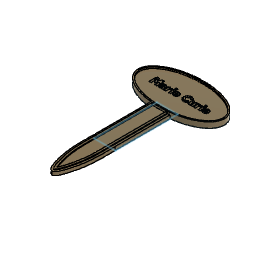
Rosen-Tafel_Marie_Curie v2 (Autodesk Fusion 360 design; units mm, degrees)
Autodesk Fusion 360 part; units mm, degrees
sketch "Skizze1" plane through (0, 0, 0) normal (0, 0, 1) x (1, 0, 0) in component "Tafe"
  ellipse E0 centre (0, 0) end of major axis (60, 0) minor radius 30
  line L0 (-60, 0) -> (60, 0)
  line L1 (0, -30) -> (0, 30)
  dimension "d1" = 60
  constraint coincident E0.centre origin
  constraint horizontal L0
  constraint coincident E0 L0.start
  constraint coincident E0 L0.end
  constraint coincident E0 L1.start
  constraint coincident E0 L1.end
  measures "d1" distance of E0
extrude "Extrusion1" add sketch "Skizze1" along normal blind 3 makes body 1 in component "Tafe"
sketch "Skizze2" plane through (0, 0, 3) normal (0, 0, 1) x (-1, 0, 0) in component "Tafe"
  ellipse E0 centre (0, 0) end of major axis (-60, 0) minor radius 30
  spline S0 degree 3 poles (61.9509, 0) (61.9509, 4.2635) (60.3055, 8.4828) (57.3091, 12.2636) (52.6449, 18.1488) (44.7166, 23.0684) (34.8255, 26.4973) (25.2136, 29.8294) (13.7584, 31.7256) (2.1658, 31.9316) (-9.8896, 32.1459) (-22.0459, 30.5274) (-32.3487, 27.3124) (-41.3637, 24.4992) (-48.9522, 20.4892) (-54.1681, 15.6411) (-58.1005, 11.9859) (-60.7028, 7.8251) (-61.5993, 3.4465) (-62.4053, -0.4903) (-61.7899, -4.5541) (-59.8722, -8.3093) (-56.3973, -15.1137) (-48.7697, -20.9418) (-38.5998, -25.0786) (-29.6788, -28.7075) (-18.796, -31.0188) (-7.5068, -31.7189) (4.0223, -32.434) (15.9353, -31.462) (26.4461, -28.9362) (36.7725, -26.4548) (45.7187, -22.4959) (52.0049, -17.4981) (56.4978, -13.926) (59.6597, -9.8063) (61.0885, -5.3839) (61.6588, -3.6187) (61.9509, -1.8099) (61.9509, 0) knots -3.141593 -3.141593 -3.141593 -3.141593 -2.764311 -2.764311 -2.764311 -2.177028 -2.177028 -2.177028 -1.606323 -1.606323 -1.606323 -1.012833 -1.012833 -1.012833 -0.49353 -0.49353 -0.49353 -0.102016 -0.102016 -0.102016 0.249996 0.249996 0.249996 0.887852 0.887852 0.887852 1.447382 1.447382 1.447382 2.018805 2.018805 2.018805 2.580199 2.580199 2.580199 2.981436 2.981436 2.981436 3.141593 3.141593 3.141593 3.141593
  dimension "d4" = 1.9509
extrude "Extrusion2" add sketch "Skizze2" along normal blind 2 and the other way blind 2 bodies 1 in component "Tafe"
sketch "Skizze3" plane through (0, 0, 0) normal (0, 0, 1) x (1, 0, 0) in component "Tafe"
extrude "Extrusion3" add 1 faces at (23.0091, -28.1834, 1) along direction (0, 0, -1) blind 1 on bodies 1 bodies 1 in component "Tafe"
sketch "Skizze1 (2)" plane through (0, 0, 0) normal (0, 0, 1) x (1, 0, 0) in component "Ständer"
extrude "Extrusion4" add 2 faces at (23.0091, -28.1834, 0) (8.4972, -9.7981, 0) along direction (0, 0, -1) blind 3 on bodies 1 bodies 1 in component "Tafe"
sketch "Skizze2 (2)" plane through (0, 0, -3) normal (0, 0, -1) x (1, 0, 0) in component "Ständer"
  spline S0 degree 3 poles (-61.9509, 0) (-61.9509, -1.8099) (-61.6588, -3.6187) (-61.0885, -5.3839) (-59.6597, -9.8063) (-56.4978, -13.926) (-52.0049, -17.4981) (-45.7187, -22.4959) (-36.7725, -26.4548) (-26.4461, -28.9362) (-15.9353, -31.462) (-4.0223, -32.434) (7.5068, -31.7189) (18.796, -31.0188) (29.6788, -28.7075) (38.5998, -25.0786) (48.7697, -20.9418) (56.3973, -15.1137) (59.8722, -8.3093) (61.7899, -4.5541) (62.4053, -0.4903) (61.5993, 3.4465) (60.7028, 7.8251) (58.1005, 11.9859) (54.1681, 15.6411) (48.9522, 20.4892) (41.3637, 24.4992) (32.3487, 27.3124) (22.0459, 30.5274) (9.8896, 32.1459) (-2.1658, 31.9316) (-13.7584, 31.7256) (-25.2136, 29.8294) (-34.8255, 26.4973) (-44.7166, 23.0684) (-52.6449, 18.1488) (-57.3091, 12.2636) (-60.3055, 8.4828) (-61.9509, 4.2635) (-61.9509, 0) knots -3.141593 -3.141593 -3.141593 -3.141593 -2.981436 -2.981436 -2.981436 -2.580199 -2.580199 -2.580199 -2.018805 -2.018805 -2.018805 -1.447382 -1.447382 -1.447382 -0.887852 -0.887852 -0.887852 -0.249996 -0.249996 -0.249996 0.102016 0.102016 0.102016 0.49353 0.49353 0.49353 1.012833 1.012833 1.012833 1.606323 1.606323 1.606323 2.177028 2.177028 2.177028 2.764311 2.764311 2.764311 3.141593 3.141593 3.141593 3.141593
  line L0 (15, 20) -> (-15, 20)
  line L1 (-15, 20) -> (-15, 110)
  line L2 (-15, 110) -> (15, 110)
  line L3 (15, 110) -> (15, 20)
  constraint horizontal L0
  constraint vertical L1
  constraint horizontal L2
  constraint vertical L3
extrude "Extrusion1'" add sketch "Skizze2 (2)" against normal blind 5 separate body contours S0 L0 L1 L3 picked at (1.6815, 23.9477) makes body 2 in component "Ständer"
extrude "Extrusion2'" add sketch "Skizze2 (2)" against normal blind 5 contours S0 L1 L2 L3 bodies 2 in component "Ständer"
sketch "Skizze3 (2)" plane through (0, 0, 2) normal (0, 0, 1) x (-1, 0, 0) in component "Ständer"
  line L0 (15, 20) -> (15, 110)
  line L1 (15, 110) -> (-15, 110)
  line L2 (-15, 110) -> (-15, 20)
  line L3 (-15, 20) -> (15, 20)
  spline S0 degree 5 poles (15, 110) (15.0176, 110.8619) (15.0503, 112.5708) (15.0915, 115.0899) (15.1309, 118.3598) (15.1537, 122.2987) (15.1484, 126.0898) (15.1122, 129.7366) (15.0406, 133.2467) (14.9275, 136.6331) (14.7639, 139.9163) (14.5397, 143.1226) (14.2439, 146.2818) (13.867, 149.4242) (13.4012, 152.5784) (12.8426, 155.769) (12.1915, 159.0132) (11.4507, 162.3163) (10.6251, 165.6668) (9.72, 169.0317) (8.7408, 172.3517) (7.6913, 175.5347) (6.574, 178.4677) (5.3908, 181.0335) (4.1426, 183.1253) (2.8302, 184.6621) (1.7296, 185.4171) (0.8758, 185.7125) (0.294, 185.7893) (0, 185.7977) knots 0 0 0 0 0 0 0.04 0.08 0.12 0.16 0.2 0.24 0.28 0.32 0.36 0.4 0.44 0.48 0.52 0.56 0.6 0.64 0.68 0.72 0.76 0.8 0.84 0.88 0.92 0.96 1 1 1 1 1 1
  line L4 (0, -2.5) -> (0, -20)
  spline S1 degree 5 poles (-15, 110) (-15.0176, 110.8619) (-15.0503, 112.5708) (-15.0915, 115.0899) (-15.1309, 118.3598) (-15.1537, 122.2987) (-15.1484, 126.0898) (-15.1122, 129.7366) (-15.0406, 133.2467) (-14.9275, 136.6331) (-14.7639, 139.9163) (-14.5397, 143.1226) (-14.2439, 146.2818) (-13.867, 149.4242) (-13.4012, 152.5784) (-12.8426, 155.769) (-12.1915, 159.0132) (-11.4507, 162.3163) (-10.6251, 165.6668) (-9.72, 169.0317) (-8.7408, 172.3517) (-7.6913, 175.5347) (-6.574, 178.4677) (-5.3908, 181.0335) (-4.1426, 183.1253) (-2.8302, 184.6621) (-1.7296, 185.4171) (-0.8758, 185.7125) (-0.294, 185.7893) (0, 185.7977) knots 0 0 0 0 0 0 0.04 0.08 0.12 0.16 0.2 0.24 0.28 0.32 0.36 0.4 0.44 0.48 0.52 0.56 0.6 0.64 0.68 0.72 0.76 0.8 0.84 0.88 0.92 0.96 1 1 1 1 1 1
  line L5 (14.8117, 100.8471) -> (15.1883, 119.1529)
  line L6 (6.7737, 185.6047) -> (-6.7737, 185.9906)
  line L7 (-14.8117, 100.8471) -> (-15.1883, 119.1529)
  line L8 (-6.7737, 185.6047) -> (6.7737, 185.9906)
  point P0 (15, 134.2579)
  point P1 (13.5579, 151.4378)
  point P2 (9.54, 169.5876)
  point P3 (3.9981, 183.1652)
  point P4 (-15, 134.2579)
  point P5 (-13.5579, 151.4378)
  point P6 (-9.54, 169.5876)
  point P7 (-3.9981, 183.1652)
  constraint coincident L0.end L1.start
  constraint midpoint L0.end L5
  constraint midpoint S0.end L6
  constraint symmetric L0.end L4 L1.end
  constraint symmetric P0 L4 P4
  constraint symmetric P1 L4 P5
  constraint symmetric P2 L4 P6
  constraint symmetric P3 L4 P7
  constraint symmetric S0.end L4 S1.end
  constraint symmetric L4 L5.start L7.start
  constraint symmetric L4 L5.end L7.end
  constraint symmetric L4 L6.start L8.start
  constraint symmetric L4 L6.end L8.end
extrude "Extrusion3'" add sketch "Skizze3 (2)" against normal blind 5 contours L1 S0 S1 bodies 2 in component "Ständer"
sketch "Skizze4" plane through (0, 0, 2) normal (0, 0, 1) x (-1, 0, 0) in component "Ständer"
  line L0 (15, 20) -> (15, 110)
  spline S0 degree 5 poles (15, 110) (15.0176, 110.8619) (15.0503, 112.5708) (15.0915, 115.0899) (15.1309, 118.3598) (15.1537, 122.2987) (15.1484, 126.0898) (15.1122, 129.7366) (15.0406, 133.2467) (14.9275, 136.6331) (14.7639, 139.9163) (14.5397, 143.1226) (14.2439, 146.2818) (13.867, 149.4242) (13.4012, 152.5784) (12.8426, 155.769) (12.1915, 159.0132) (11.4507, 162.3163) (10.6251, 165.6668) (9.72, 169.0317) (8.7408, 172.3517) (7.6913, 175.5347) (6.574, 178.4677) (5.3908, 181.0335) (4.1426, 183.1253) (2.8302, 184.6621) (1.7296, 185.4171) (0.8758, 185.7125) (0.294, 185.7893) (0, 185.7977) knots 0 0 0 0 0 0 0.04 0.08 0.12 0.16 0.2 0.24 0.28 0.32 0.36 0.4 0.44 0.48 0.52 0.56 0.6 0.64 0.68 0.72 0.76 0.8 0.84 0.88 0.92 0.96 1 1 1 1 1 1
  spline S1 degree 5 poles (-15, 110) (-15.0176, 110.8619) (-15.0503, 112.5708) (-15.0915, 115.0899) (-15.1309, 118.3598) (-15.1537, 122.2987) (-15.1484, 126.0898) (-15.1122, 129.7366) (-15.0406, 133.2467) (-14.9275, 136.6331) (-14.7639, 139.9163) (-14.5397, 143.1226) (-14.2439, 146.2818) (-13.867, 149.4242) (-13.4012, 152.5784) (-12.8426, 155.769) (-12.1915, 159.0132) (-11.4507, 162.3163) (-10.6251, 165.6668) (-9.72, 169.0317) (-8.7408, 172.3517) (-7.6913, 175.5347) (-6.574, 178.4677) (-5.3908, 181.0335) (-4.1426, 183.1253) (-2.8302, 184.6621) (-1.7296, 185.4171) (-0.8758, 185.7125) (-0.294, 185.7893) (0, 185.7977) knots 0 0 0 0 0 0 0.04 0.08 0.12 0.16 0.2 0.24 0.28 0.32 0.36 0.4 0.44 0.48 0.52 0.56 0.6 0.64 0.68 0.72 0.76 0.8 0.84 0.88 0.92 0.96 1 1 1 1 1 1
  line L1 (-15, 110) -> (-15, 20)
  line L2 (-15, 20) -> (15, 20)
  spline S2 degree 3 poles (-11.9777, 110.0309) (-11.9779, 110.0412) (-11.9781, 110.0515) (-11.9783, 110.0618) (-12.1467, 118.2962) (-12.1876, 125.6884) (-12.0304, 132.2915) (-11.8915, 138.1249) (-11.5879, 143.3276) (-10.915, 148.5264) (-10.4464, 152.1476) (-9.7926, 155.8041) (-8.949, 159.6156) (-8.1726, 163.1233) (-7.2391, 166.7794) (-6.1929, 170.2595) (-5.0109, 174.1918) (-3.6533, 177.8638) (-2.3593, 180.1318) (-1.7058, 181.2772) (-1.0734, 182.0403) (-0.6357, 182.4064) (-0.297, 182.6897) (-0.1153, 182.7456) (0, 182.7673) knots -0.000287 -0.000287 -0.000287 -0.000287 0 0 0 0.23016 0.23016 0.23016 0.433487 0.433487 0.433487 0.575116 0.575116 0.575116 0.705456 0.705456 0.705456 0.852728 0.852728 0.852728 0.927106 0.927106 0.927106 0.984664 0.984664 0.984664 0.984664
  spline S3 degree 3 poles (11.9777, 110.0309) (11.9779, 110.0412) (11.9781, 110.0515) (11.9783, 110.0618) (12.1467, 118.2962) (12.1876, 125.6884) (12.0304, 132.2915) (11.8915, 138.1249) (11.5879, 143.3276) (10.915, 148.5264) (10.4464, 152.1476) (9.7926, 155.8041) (8.949, 159.6156) (8.1726, 163.1233) (7.2391, 166.7794) (6.1929, 170.2595) (5.0109, 174.1918) (3.6533, 177.8638) (2.3593, 180.1318) (1.7058, 181.2772) (1.0734, 182.0403) (0.6357, 182.4064) (0.297, 182.6897) (0.1153, 182.7456) (0, 182.7673) knots -0.000287 -0.000287 -0.000287 -0.000287 0 0 0 0.23016 0.23016 0.23016 0.433487 0.433487 0.433487 0.575116 0.575116 0.575116 0.705456 0.705456 0.705456 0.852728 0.852728 0.852728 0.927106 0.927106 0.927106 0.984664 0.984664 0.984664 0.984664
  line L3 (11.9777, 23.0223) -> (11.9777, 110.0309)
  line L4 (-11.9777, 23.0223) -> (11.9777, 23.0223)
  line L5 (-11.9777, 110.0309) -> (-11.9777, 23.0223)
  spline S4 degree 3 poles (-9, 110.0613) (-9.0004, 110.0818) (-9.0008, 110.1022) (-9.0013, 110.1226) (-9.1708, 118.4153) (-9.2103, 125.8461) (-9.0484, 132.4316) (-8.9146, 137.8751) (-8.6346, 142.7164) (-8.0427, 147.5055) (-7.6174, 150.9474) (-7.0241, 154.4041) (-6.2475, 158.0272) (-5.5493, 161.2843) (-4.705, 164.6878) (-3.7598, 167.9778) (-2.8347, 171.1978) (-1.801, 174.2968) (-0.8034, 176.5706) (-0.5276, 177.1992) (-0.2561, 177.763) (0, 178.2439) knots -0.000569 -0.000569 -0.000569 -0.000569 0 0 0 0.232641 0.232641 0.232641 0.424939 0.424939 0.424939 0.56314 0.56314 0.56314 0.687378 0.687378 0.687378 0.80897 0.80897 0.80897 0.842587 0.842587 0.842587 0.842587
  spline S5 degree 3 poles (9, 110.0613) (9.0004, 110.0818) (9.0008, 110.1022) (9.0013, 110.1226) (9.1708, 118.4153) (9.2103, 125.8461) (9.0484, 132.4316) (8.9146, 137.8751) (8.6346, 142.7164) (8.0427, 147.5055) (7.6174, 150.9474) (7.0241, 154.4041) (6.2475, 158.0272) (5.5493, 161.2843) (4.705, 164.6878) (3.7598, 167.9778) (2.8347, 171.1978) (1.801, 174.2968) (0.8034, 176.5706) (0.5276, 177.1992) (0.2561, 177.763) (0, 178.2439) knots -0.000569 -0.000569 -0.000569 -0.000569 0 0 0 0.232641 0.232641 0.232641 0.424939 0.424939 0.424939 0.56314 0.56314 0.56314 0.687378 0.687378 0.687378 0.80897 0.80897 0.80897 0.842587 0.842587 0.842587 0.842587
  line L6 (9, 26) -> (9, 110.0613)
  line L7 (-9, 26) -> (9, 26)
  line L8 (-9, 110.0613) -> (-9, 26)
  dimension "d19" = -3.0223
  dimension "d20" = -6
extrude "Extrusion4'" add sketch "Skizze4" along normal blind 1 contours S2 S3 L3 L4 L5 bodies 2 in component "Ständer"
combine "Kombinieren1" operation add target body 1 tool bodies 2 in component "Tafe"
sketch "Skizze1 (3)" plane through (0, 0, 3) normal (0, 0, 1) x (-1, 0, 0)
  ellipse E0 centre (0, 0) end of major axis (-60, 0) minor radius 30
  line L0 (37.6827, 1.5082) -> (37.6827, 5.3738)
  line L1 (37.6827, 5.3738) -> (40.7098, 5.3738)
  line L2 (40.7098, 5.3738) -> (40.7098, -3.8782)
  line L3 (40.7098, -3.8782) -> (37.6827, 1.5082)
  line L4 (40.2977, -5.6262) -> (37.2095, -5.6262)
  line L5 (37.2095, -5.6262) -> (35.1032, -1.4621)
  line L6 (35.1032, -1.4621) -> (32.8833, -5.6262)
  line L7 (32.8833, -5.6262) -> (29.4256, -5.6262)
  line L8 (29.4256, -5.6262) -> (29.4256, 5.3738)
  line L9 (29.4256, 5.3738) -> (32.5238, 5.3738)
  line L10 (32.5238, 5.3738) -> (32.5238, -1.0074)
  line L11 (32.5238, -1.0074) -> (35.1032, 3.5831)
  line L12 (35.1032, 3.5831) -> (40.2977, -5.6262)
  spline S0 degree 2 poles (25.56, -0.4105) (26.3132, -0.3536) (26.7822, -0.2044) knots 0 0 0 1 1 1
  spline S1 degree 2 poles (26.7822, -0.2044) (27.2512, -0.0552) (27.5354, 0.1012) knots 0 0 0 1 1 1
  line L13 (27.5354, 0.1012) -> (28.2602, -1.6753)
  spline S2 degree 2 poles (28.2602, -1.6753) (27.8481, -1.8743) (27.2156, -2.0519) knots 0 0 0 1 1 1
  spline S3 degree 2 poles (27.2156, -2.0519) (26.5832, -2.2296) (25.56, -2.3148) knots 0 0 0 1 1 1
  line L14 (25.56, -2.3148) -> (25.56, -0.4105)
  spline S4 degree 2 poles (24.7214, 1.9771) (25.2899, 1.9914) (25.6168, 2.2543) knots 0 0 0 1 1 1
  spline S5 degree 2 poles (25.6168, 2.2543) (25.9437, 2.5172) (25.9437, 2.972) knots 0 0 0 1 1 1
  spline S6 degree 2 poles (25.9437, 2.972) (25.9437, 3.4125) (25.5671, 3.6186) knots 0 0 0 1 1 1
  spline S7 degree 2 poles (25.5671, 3.6186) (25.1904, 3.8247) (24.7214, 3.8389) knots 0 0 0 1 1 1
  line L15 (24.7214, 3.8389) -> (24.7214, 5.388)
  spline S8 degree 2 poles (24.7214, 5.388) (24.9631, 5.4591) (25.2331, 5.5017) knots 0 0 0 1 1 1
  spline S9 degree 2 poles (25.2331, 5.5017) (25.5031, 5.5443) (25.83, 5.5443) knots 0 0 0 1 1 1
  spline S10 degree 2 poles (25.83, 5.5443) (26.4553, 5.5443) (26.9882, 5.3596) knots 0 0 0 1 1 1
  spline S11 degree 2 poles (26.9882, 5.3596) (27.5212, 5.1748) (27.9049, 4.8408) knots 0 0 0 1 1 1
  spline S12 degree 2 poles (27.9049, 4.8408) (28.2886, 4.5069) (28.5089, 4.0308) knots 0 0 0 1 1 1
  spline S13 degree 2 poles (28.5089, 4.0308) (28.7292, 3.5547) (28.7292, 2.972) knots 0 0 0 1 1 1
  spline S14 degree 2 poles (28.7292, 2.972) (28.7292, 2.3324) (28.4805, 1.8563) knots 0 0 0 1 1 1
  spline S15 degree 2 poles (28.4805, 1.8563) (28.2318, 1.3802) (27.8054, 1.0534) knots 0 0 0 1 1 1
  spline S16 degree 2 poles (27.8054, 1.0534) (27.3791, 0.7265) (26.8035, 0.5631) knots 0 0 0 1 1 1
  spline S17 degree 2 poles (26.8035, 0.5631) (26.2279, 0.3996) (25.56, 0.3996) knots 0 0 0 1 1 1
  spline S18 degree 2 poles (25.56, 0.3996) (25.1904, 0.3996) (24.7214, 0.4849) knots 0 0 0 1 1 1
  line L16 (24.7214, 0.4849) -> (24.7214, 1.9771)
  spline S19 degree 2 poles (24.3235, -2.3291) (23.5134, -2.2864) (22.8384, -2.0803) knots 0 0 0 1 1 1
  spline S20 degree 2 poles (22.8384, -2.0803) (22.1633, -1.8743) (21.6801, -1.4408) knots 0 0 0 1 1 1
  spline S21 degree 2 poles (21.6801, -1.4408) (21.1969, -1.0074) (20.9269, -0.3181) knots 0 0 0 1 1 1
  spline S22 degree 2 poles (20.9269, -0.3181) (20.6568, 0.3712) (20.6568, 1.3802) knots 0 0 0 1 1 1
  line L17 (20.6568, 1.3802) -> (20.6568, 5.3738)
  line L18 (20.6568, 5.3738) -> (23.485, 5.3738)
  line L19 (23.485, 5.3738) -> (23.485, 0.5986)
  spline S23 degree 2 poles (23.485, 0.5986) (23.5134, 0.2291) (23.7266, 0.0088) knots 0 0 0 1 1 1
  spline S24 degree 2 poles (23.7266, 0.0088) (23.9398, -0.2115) (24.3235, -0.2968) knots 0 0 0 1 1 1
  line L20 (24.3235, -0.2968) -> (24.3235, -2.3291)
  spline S25 degree 2 poles (13.7357, 0.1012) (13.8636, 0.1012) (14.0625, 0.1083) knots 0 0 0 1 1 1
  spline S26 degree 2 poles (14.0625, 0.1083) (14.2615, 0.1154) (14.5031, 0.1509) knots 0 0 0 1 1 1
  spline S27 degree 2 poles (14.5031, 0.1509) (14.7447, 0.1864) (15.0005, 0.2575) knots 0 0 0 1 1 1
  spline S28 degree 2 poles (15.0005, 0.2575) (15.2563, 0.3286) (15.4837, 0.4707) knots 0 0 0 1 1 1
  line L21 (15.4837, 0.4707) -> (15.4837, -1.9738)
  spline S29 degree 2 poles (15.4837, -1.9738) (15.1853, -2.1301) (14.7589, -2.2367) knots 0 0 0 1 1 1
  spline S30 degree 2 poles (14.7589, -2.2367) (14.3326, -2.3433) (13.7357, -2.3433) knots 0 0 0 1 1 1
  line L22 (13.7357, -2.3433) -> (13.7357, 0.1012)
  line L23 (16.6917, 5.3738) -> (19.5199, 5.3738)
  line L24 (19.5199, 5.3738) -> (19.5199, -2.1727)
  line L25 (19.5199, -2.1727) -> (16.6917, -2.1727)
  line L26 (16.6917, -2.1727) -> (16.6917, 5.3738)
  line L27 (12.8687, -2.1727) -> (10.0406, -2.1727)
  line L28 (10.0406, -2.1727) -> (10.0406, 5.3738)
  line L29 (10.0406, 5.3738) -> (12.8687, 5.3738)
  line L30 (12.8687, 5.3738) -> (12.8687, -2.1727)
  line L31 (12.8687, -3.1818) -> (12.8687, -5.612)
  line L32 (12.8687, -5.612) -> (10.0406, -5.612)
  line L33 (10.0406, -5.612) -> (10.0406, -3.1818)
  line L34 (10.0406, -3.1818) -> (12.8687, -3.1818)
  line L35 (5.4643, 0.9681) -> (4.0005, 0.9681)
  spline S31 degree 2 poles (4.0005, 0.9681) (4.0005, 0.6554) (4.1426, 0.3428) knots 0 0 0 1 1 1
  spline S32 degree 2 poles (4.1426, 0.3428) (4.2848, 0.0301) (4.6258, -0.1262) knots 0 0 0 1 1 1
  line L36 (4.6258, -0.1262) -> (4.6258, -2.3148)
  spline S33 degree 2 poles (4.6258, -2.3148) (3.8584, -2.2296) (3.2402, -1.9098) knots 0 0 0 1 1 1
  spline S34 degree 2 poles (3.2402, -1.9098) (2.622, -1.59) (2.1885, -1.0713) knots 0 0 0 1 1 1
  spline S35 degree 2 poles (2.1885, -1.0713) (1.755, -0.5526) (1.5205, 0.1509) knots 0 0 0 1 1 1
  spline S36 degree 2 poles (1.5205, 0.1509) (1.286, 0.8544) (1.286, 1.7071) knots 0 0 0 1 1 1
  spline S37 degree 2 poles (1.286, 1.7071) (1.286, 1.8919) (1.3571, 2.0624) knots 0 0 0 1 1 1
  line L37 (1.3571, 2.0624) -> (5.4643, 2.0624)
  line L38 (5.4643, 2.0624) -> (5.4643, 0.9681)
  spline S38 degree 2 poles (5.8623, -0.0978) (6.1891, 0.1154) (6.3455, 0.5489) knots 0 0 0 1 1 1
  spline S39 degree 2 poles (6.3455, 0.5489) (6.5018, 0.9823) (6.5018, 1.4513) knots 0 0 0 1 1 1
  spline S40 degree 2 poles (6.5018, 1.4513) (6.5018, 1.9487) (6.3384, 2.4106) knots 0 0 0 1 1 1
  spline S41 degree 2 poles (6.3384, 2.4106) (6.1749, 2.8725) (5.8623, 3.0715) knots 0 0 0 1 1 1
  line L39 (5.8623, 3.0715) -> (5.8623, 5.5017)
  spline S42 degree 2 poles (5.8623, 5.5017) (6.6581, 5.4022) (7.2764, 5.0682) knots 0 0 0 1 1 1
  spline S43 degree 2 poles (7.2764, 5.0682) (7.8946, 4.7343) (8.3209, 4.2226) knots 0 0 0 1 1 1
  spline S44 degree 2 poles (8.3209, 4.2226) (8.7473, 3.711) (8.9747, 3.043) knots 0 0 0 1 1 1
  spline S45 degree 2 poles (8.9747, 3.043) (9.2021, 2.3751) (9.2021, 1.6076) knots 0 0 0 1 1 1
  spline S46 degree 2 poles (9.2021, 1.6076) (9.2021, 0.8402) (8.9676, 0.1722) knots 0 0 0 1 1 1
  spline S47 degree 2 poles (8.9676, 0.1722) (8.7331, -0.4957) (8.2925, -1.0074) knots 0 0 0 1 1 1
  spline S48 degree 2 poles (8.2925, -1.0074) (7.8519, -1.519) (7.2408, -1.853) knots 0 0 0 1 1 1
  spline S49 degree 2 poles (7.2408, -1.853) (6.6297, -2.1869) (5.8623, -2.3006) knots 0 0 0 1 1 1
  line L40 (5.8623, -2.3006) -> (5.8623, -0.0978)
  spline S50 degree 2 poles (1.5561, 3.7394) (1.7977, 4.18) (2.1956, 4.5211) knots 0 0 0 1 1 1
  spline S51 degree 2 poles (2.1956, 4.5211) (2.5935, 4.8622) (3.1762, 5.1464) knots 0 0 0 1 1 1
  spline S52 degree 2 poles (3.1762, 5.1464) (3.7589, 5.4306) (4.6258, 5.5159) knots 0 0 0 1 1 1
  line L41 (4.6258, 5.5159) -> (4.6258, 3.2562)
  spline S53 degree 2 poles (4.6258, 3.2562) (4.3416, 3.1994) (4.1497, 3.0857) knots 0 0 0 1 1 1
  spline S54 degree 2 poles (4.1497, 3.0857) (3.9579, 2.972) (3.8158, 2.8441) knots 0 0 0 1 1 1
  spline S55 degree 2 poles (3.8158, 2.8441) (3.6736, 2.7162) (3.5742, 2.5598) knots 0 0 0 1 1 1
  line L42 (3.5742, 2.5598) -> (1.5561, 3.7394)
  spline S56 degree 2 poles (-9.6145, -5.9105) (-10.9362, -5.8252) (-12.0376, -5.2638) knots 0 0 0 1 1 1
  spline S57 degree 2 poles (-12.0376, -5.2638) (-13.139, -4.7024) (-13.8638, -3.736) knots 0 0 0 1 1 1
  line L43 (-13.8638, -3.736) -> (-11.4194, -1.8316)
  spline S58 degree 2 poles (-11.4194, -1.8316) (-11.1351, -2.2864) (-10.6448, -2.5422) knots 0 0 0 1 1 1
  spline S59 degree 2 poles (-10.6448, -2.5422) (-10.1545, -2.798) (-9.6145, -2.8833) knots 0 0 0 1 1 1
  line L44 (-9.6145, -2.8833) -> (-9.6145, -5.9105)
  spline S60 degree 2 poles (-8.3638, 5.6296) (-7.2411, 5.5017) (-6.3102, 5.0256) knots 0 0 0 1 1 1
  spline S61 degree 2 poles (-6.3102, 5.0256) (-5.3793, 4.5495) (-4.7185, 3.7892) knots 0 0 0 1 1 1
  spline S62 degree 2 poles (-4.7185, 3.7892) (-4.0576, 3.0288) (-3.6952, 2.034) knots 0 0 0 1 1 1
  spline S63 degree 2 poles (-3.6952, 2.034) (-3.3328, 1.0392) (-3.3328, -0.1262) knots 0 0 0 1 1 1
  spline S64 degree 2 poles (-3.3328, -0.1262) (-3.3328, -1.249) (-3.7023, -2.2367) knots 0 0 0 1 1 1
  spline S65 degree 2 poles (-3.7023, -2.2367) (-4.0718, -3.2244) (-4.7398, -3.9847) knots 0 0 0 1 1 1
  spline S66 degree 2 poles (-4.7398, -3.9847) (-5.4077, -4.7451) (-6.3315, -5.2425) knots 0 0 0 1 1 1
  spline S67 degree 2 poles (-6.3315, -5.2425) (-7.2553, -5.7399) (-8.3638, -5.8678) knots 0 0 0 1 1 1
  line L45 (-8.3638, -5.8678) -> (-8.3638, -2.798)
  spline S68 degree 2 poles (-8.3638, -2.798) (-7.5111, -2.5564) (-6.9782, -1.853) knots 0 0 0 1 1 1
  spline S69 degree 2 poles (-6.9782, -1.853) (-6.4452, -1.1495) (-6.4452, -0.1262) knots 0 0 0 1 1 1
  spline S70 degree 2 poles (-6.4452, -0.1262) (-6.4452, 0.3286) (-6.5873, 0.7549) knots 0 0 0 1 1 1
  spline S71 degree 2 poles (-6.5873, 0.7549) (-6.7295, 1.1813) (-6.9853, 1.5295) knots 0 0 0 1 1 1
  spline S72 degree 2 poles (-6.9853, 1.5295) (-7.2411, 1.8777) (-7.5964, 2.1406) knots 0 0 0 1 1 1
  spline S73 degree 2 poles (-7.5964, 2.1406) (-7.9517, 2.4035) (-8.3638, 2.5314) knots 0 0 0 1 1 1
  line L46 (-8.3638, 2.5314) -> (-8.3638, 5.6296)
  spline S74 degree 2 poles (-13.9065, 3.2562) (-13.2101, 4.3079) (-12.1015, 4.9332) knots 0 0 0 1 1 1
  spline S75 degree 2 poles (-12.1015, 4.9332) (-10.993, 5.5585) (-9.6145, 5.658) knots 0 0 0 1 1 1
  line L47 (-9.6145, 5.658) -> (-9.6145, 2.6025)
  spline S76 degree 2 poles (-9.6145, 2.6025) (-10.1403, 2.4888) (-10.588, 2.1761) knots 0 0 0 1 1 1
  spline S77 degree 2 poles (-10.588, 2.1761) (-11.0357, 1.8634) (-11.3199, 1.4087) knots 0 0 0 1 1 1
  line L48 (-11.3199, 1.4087) -> (-13.9065, 3.2562)
  line L49 (-19.0796, -2.1727) -> (-21.8651, -2.1727)
  line L50 (-21.8651, -2.1727) -> (-21.8651, 5.3738)
  line L51 (-21.8651, 5.3738) -> (-19.0796, 5.3738)
  line L52 (-19.0796, 5.3738) -> (-19.0796, -2.1727)
  spline S78 degree 2 poles (-17.8858, 5.2885) (-17.6158, 5.4022) (-17.2889, 5.4733) knots 0 0 0 1 1 1
  spline S79 degree 2 poles (-17.2889, 5.4733) (-16.962, 5.5443) (-16.5641, 5.5443) knots 0 0 0 1 1 1
  spline S80 degree 2 poles (-16.5641, 5.5443) (-15.4413, 5.5443) (-14.9155, 4.9048) knots 0 0 0 1 1 1
  spline S81 degree 2 poles (-14.9155, 4.9048) (-14.3897, 4.2653) (-14.3897, 3.2278) knots 0 0 0 1 1 1
  line L53 (-14.3897, 3.2278) -> (-14.3897, -2.1727)
  line L54 (-14.3897, -2.1727) -> (-17.2889, -2.1727)
  line L55 (-17.2889, -2.1727) -> (-17.2889, 1.8919)
  spline S82 degree 2 poles (-17.2889, 1.8919) (-17.2889, 2.6167) (-17.4026, 2.8654) knots 0 0 0 1 1 1
  spline S83 degree 2 poles (-17.4026, 2.8654) (-17.5163, 3.1141) (-17.8858, 3.1709) knots 0 0 0 1 1 1
  line L56 (-17.8858, 3.1709) -> (-17.8858, 5.2885)
  spline S84 degree 2 poles (-28.7437, 0.1012) (-28.6158, 0.1012) (-28.4168, 0.1083) knots 0 0 0 1 1 1
  spline S85 degree 2 poles (-28.4168, 0.1083) (-28.2178, 0.1154) (-27.9762, 0.1509) knots 0 0 0 1 1 1
  spline S86 degree 2 poles (-27.9762, 0.1509) (-27.7346, 0.1864) (-27.4788, 0.2575) knots 0 0 0 1 1 1
  spline S87 degree 2 poles (-27.4788, 0.2575) (-27.223, 0.3286) (-26.9956, 0.4707) knots 0 0 0 1 1 1
  line L57 (-26.9956, 0.4707) -> (-26.9956, -1.9738)
  spline S88 degree 2 poles (-26.9956, -1.9738) (-27.2941, -2.1301) (-27.7204, -2.2367) knots 0 0 0 1 1 1
  spline S89 degree 2 poles (-27.7204, -2.2367) (-28.1468, -2.3433) (-28.7437, -2.3433) knots 0 0 0 1 1 1
  line L58 (-28.7437, -2.3433) -> (-28.7437, 0.1012)
  line L59 (-25.7876, 5.3738) -> (-22.9594, 5.3738)
  line L60 (-22.9594, 5.3738) -> (-22.9594, -2.1727)
  line L61 (-22.9594, -2.1727) -> (-25.7876, -2.1727)
  line L62 (-25.7876, -2.1727) -> (-25.7876, 5.3738)
  line L63 (-29.6106, -2.1727) -> (-32.4388, -2.1727)
  line L64 (-32.4388, -2.1727) -> (-32.4388, 5.3738)
  line L65 (-32.4388, 5.3738) -> (-29.6106, 5.3738)
  line L66 (-29.6106, 5.3738) -> (-29.6106, -2.1727)
  line L67 (-29.6106, -3.1818) -> (-29.6106, -5.612)
  line L68 (-29.6106, -5.612) -> (-32.4388, -5.612)
  line L69 (-32.4388, -5.612) -> (-32.4388, -3.1818)
  line L70 (-32.4388, -3.1818) -> (-29.6106, -3.1818)
  line L71 (-37.015, 0.9681) -> (-38.4788, 0.9681)
  spline S90 degree 2 poles (-38.4788, 0.9681) (-38.4788, 0.6554) (-38.3367, 0.3428) knots 0 0 0 1 1 1
  spline S91 degree 2 poles (-38.3367, 0.3428) (-38.1946, 0.0301) (-37.8535, -0.1262) knots 0 0 0 1 1 1
  line L72 (-37.8535, -0.1262) -> (-37.8535, -2.3148)
  spline S92 degree 2 poles (-37.8535, -2.3148) (-38.6209, -2.2296) (-39.2392, -1.9098) knots 0 0 0 1 1 1
  spline S93 degree 2 poles (-39.2392, -1.9098) (-39.8574, -1.59) (-40.2908, -1.0713) knots 0 0 0 1 1 1
  spline S94 degree 2 poles (-40.2908, -1.0713) (-40.7243, -0.5526) (-40.9588, 0.1509) knots 0 0 0 1 1 1
  spline S95 degree 2 poles (-40.9588, 0.1509) (-41.1933, 0.8544) (-41.1933, 1.7071) knots 0 0 0 1 1 1
  spline S96 degree 2 poles (-41.1933, 1.7071) (-41.1933, 1.8919) (-41.1222, 2.0624) knots 0 0 0 1 1 1
  line L73 (-41.1222, 2.0624) -> (-37.015, 2.0624)
  line L74 (-37.015, 2.0624) -> (-37.015, 0.9681)
  spline S97 degree 2 poles (-36.6171, -0.0978) (-36.2902, 0.1154) (-36.1338, 0.5489) knots 0 0 0 1 1 1
  spline S98 degree 2 poles (-36.1338, 0.5489) (-35.9775, 0.9823) (-35.9775, 1.4513) knots 0 0 0 1 1 1
  spline S99 degree 2 poles (-35.9775, 1.4513) (-35.9775, 1.9487) (-36.141, 2.4106) knots 0 0 0 1 1 1
  spline S100 degree 2 poles (-36.141, 2.4106) (-36.3044, 2.8725) (-36.6171, 3.0715) knots 0 0 0 1 1 1
  line L75 (-36.6171, 3.0715) -> (-36.6171, 5.5017)
  spline S101 degree 2 poles (-36.6171, 5.5017) (-35.8212, 5.4022) (-35.203, 5.0682) knots 0 0 0 1 1 1
  spline S102 degree 2 poles (-35.203, 5.0682) (-34.5848, 4.7343) (-34.1584, 4.2226) knots 0 0 0 1 1 1
  spline S103 degree 2 poles (-34.1584, 4.2226) (-33.732, 3.711) (-33.5047, 3.043) knots 0 0 0 1 1 1
  spline S104 degree 2 poles (-33.5047, 3.043) (-33.2773, 2.3751) (-33.2773, 1.6076) knots 0 0 0 1 1 1
  spline S105 degree 2 poles (-33.2773, 1.6076) (-33.2773, 0.8402) (-33.5118, 0.1722) knots 0 0 0 1 1 1
  spline S106 degree 2 poles (-33.5118, 0.1722) (-33.7463, -0.4957) (-34.1868, -1.0074) knots 0 0 0 1 1 1
  spline S107 degree 2 poles (-34.1868, -1.0074) (-34.6274, -1.519) (-35.2385, -1.853) knots 0 0 0 1 1 1
  spline S108 degree 2 poles (-35.2385, -1.853) (-35.8496, -2.1869) (-36.6171, -2.3006) knots 0 0 0 1 1 1
  line L76 (-36.6171, -2.3006) -> (-36.6171, -0.0978)
  spline S109 degree 2 poles (-40.9233, 3.7394) (-40.6817, 4.18) (-40.2837, 4.5211) knots 0 0 0 1 1 1
  spline S110 degree 2 poles (-40.2837, 4.5211) (-39.8858, 4.8622) (-39.3031, 5.1464) knots 0 0 0 1 1 1
  spline S111 degree 2 poles (-39.3031, 5.1464) (-38.7204, 5.4306) (-37.8535, 5.5159) knots 0 0 0 1 1 1
  line L77 (-37.8535, 5.5159) -> (-37.8535, 3.2562)
  spline S112 degree 2 poles (-37.8535, 3.2562) (-38.1377, 3.1994) (-38.3296, 3.0857) knots 0 0 0 1 1 1
  spline S113 degree 2 poles (-38.3296, 3.0857) (-38.5214, 2.972) (-38.6636, 2.8441) knots 0 0 0 1 1 1
  spline S114 degree 2 poles (-38.6636, 2.8441) (-38.8057, 2.7162) (-38.9052, 2.5598) knots 0 0 0 1 1 1
  line L78 (-38.9052, 2.5598) -> (-40.9233, 3.7394)
extrude "Extrusion5" cut sketch "Skizze1 (3)" against normal blind 20 contours L0 L1 L2 L3 | L4 L5 L6 L7 L8 L9 L10 L11 L12 | S0 S1 L13 S2 S3 L14 | S4 S5 S6 S7 L15 S8 S9 S10 S11 S12 S13 S14 S15 S16 S17 S18 L16 | S19 S20 S21 S22 L17 L18 L19 S23 S24 L20 | S25 S26 S27 S28 L21 S29 S30 L22 | L23 L24 L25 L26 | L27 L28 L29 L30 | L31 L32 L33 L34 | L35 S31 S32 L36 S33 S34 S35 S36 S37 L37 L38 | S38 S39 S40 S41 L39 S42 S43 S44 S45 S46 S47 S48 S49 L40 | S50 S51 S52 L41 S53 S54 S55 L42 | S56 S57 L43 S58 S59 L44 | S60 S61 S62 S63 S64 S65 S66 S67 L45 S68 S69 S70 S71 S72 S73 L46 | S74 S75 L47 S76 S77 L48 | L49 L50 L51 L52 | S78 S79 S80 S81 L53 L54 L55 S82 S83 L56 | S84 S85 S86 S87 L57 S88 S89 L58 | L59 L60 L61 L62 | L63 L64 L65 L66 | L67 L68 L69 L70 | L71 S90 S91 L72 S92 S93 S94 S95 S96 L73 L74 | S97 S98 S99 S100 L75 S101 S102 S103 S104 S105 S106 S107 S108 L76 | S109 S110 S111 L77 S112 S113 S114 L78 bodies 1 in component "Tafe"
component "Tafe" placed x (1, 0, 0) y (0, 1, 0) z (0, 0, 1) at (0, 0, 0)
component "Ständer" placed x (1, 0, 0) y (0, 1, 0) z (0, 0, 1) at (0, 0, 0)
named bodies: "Grundplatte"
